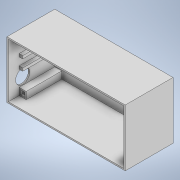
# Autodesk Inventor part: TimBoden
Saved by Autodesk Inventor 2022 (Build 260153000, 153)
## iProperties
Created: 2023-01-01
Part Number: TimBoden
Material: Generisch
Document SubType Name: Modeling
Designer: Joshua
Density: 1 g/cm^3
Appearance: Vorgabe
Author: Joshua
Autodesk Inventor part; units mm, degrees
ref_plane "YZ Plane" through (0, 0, 0) normal (1, 0, 0) x (0, 1, 0)
ref_plane "XZ Plane" through (0, 0, 0) normal (0, 1, 0) x (-1, 0, 0)
ref_plane "XY Plane" through (0, 0, 0) normal (0, 0, 1) x (1, 0, 0)
sketch "Skizze1" plane through (0, 0, 0) normal (0, 0, 1) x (1, 0, 0)
  line L0 (0, 0) -> (166, 0)
  line L1 (166, 0) -> (166, 80)
  line L2 (166, 80) -> (0, 80)
  line L3 (0, 80) -> (0, 0)
  dimension "d0" = 80
  dimension "d1" = 166
  constraints: 8 end point, 2 parallel, 1 horizontal, 1 perpendicular
  measures "d0" distance of L2.end L0.start
  measures "d1" distance of L1.end L2.end
extrude "Extrusion1" add sketch "Skizze1" along normal blind 2
sketch "Skizze2" plane through (0, 0, 2) normal (0, 0, 1) x (1, 0, 0)
  line L0 (0, 80) -> (0, 0) projected
  line L1 (166, 0) -> (166, 80) projected
  line L2 (0, 0) -> (166, 0)
  line L3 (166, 0) -> (166, 80)
  line L4 (166, 80) -> (0, 80)
  line L5 (0, 80) -> (0, 0)
  line L6 (2, 78) -> (164, 78)
  line L7 (164, 78) -> (164, 2)
  line L8 (164, 2) -> (2, 2)
  line L9 (2, 2) -> (2, 78)
  dimension "d4" = 2
  dimension "d6" = 2
  dimension "d7" = 2
  dimension "d8" = 2
  constraints: 16 end point, 4 parallel, 2 horizontal, 2 perpendicular
  measures "d4" distance between parallel lines of L0 L9
  measures "d6" distance between parallel lines of L4 L6
  measures "d7" distance between parallel lines of L1 L7
  measures "d8" distance between parallel lines of L2 L8
extrude "Extrusion2" add sketch "Skizze2" along normal blind 65
sketch "Skizze4" plane through (0, 0, 2) normal (0, 0, 1) x (1, 0, 0)
  line L0 (2, 2) -> (2, 78) projected
  line L1 (164, 2) -> (2, 2) projected
  line L2 (2, 78) -> (164, 78)
  line L3 (164, 78) -> (164, 2)
  line L4 (164, 2) -> (2, 2)
  line L5 (2, 2) -> (2, 78)
  line L6 (2, 68) -> (12, 68)
  line L7 (12, 68) -> (12, 78)
  line L8 (12, 78) -> (2, 78)
  line L9 (2, 78) -> (2, 68)
  line L10 (2, 2) -> (12, 2)
  line L11 (12, 2) -> (12, 12)
  line L12 (12, 12) -> (2, 12)
  line L13 (2, 12) -> (2, 2)
  line L14 (164, 78) -> (164, 2) projected
  line L15 (2, 78) -> (164, 78) projected
  line L16 (164, 68) -> (154, 68)
  line L17 (154, 68) -> (154, 78)
  line L18 (154, 78) -> (164, 78)
  line L19 (164, 78) -> (164, 68)
  line L20 (164, 2) -> (154, 2)
  line L21 (154, 2) -> (154, 12)
  line L22 (154, 12) -> (164, 12)
  line L23 (164, 12) -> (164, 2)
  point P0 (0, 0)
  point P1 (164, 12)
  point P2 (12, 2)
  point P3 (2, 68)
  dimension "d20" = 10
  dimension "d21" = 10
  dimension "d22" = 10
  dimension "d23" = 10
  dimension "d41" = 10
  dimension "d55" = 10
  constraints: 40 end point, 10 parallel, 5 horizontal, 5 perpendicular, 4 point on line
  measures "d20" distance of L6.end L7.end
  measures "d21" distance of L6.start L6.end
  measures "d22" distance of L10.end L11.end
  measures "d23" distance of L16.start L16.end
  measures "d41" distance of L11.end L12.end
  measures "d55" distance of L16.end L17.end
extrude "Extrusion3" add sketch "Skizze4" along normal blind 50 contours L0 L12 L11 L1 | L0 L2 L7 L6 | L21 L22 L3 L1 | L2 L3 L16 L17
sketch "Skizze5" plane through (0, 0, 2) normal (0, 0, 1) x (1, 0, 0)
  line L0 (2, 78) -> (164, 78) projected
  line L1 (2, 2) -> (2, 78) projected
  line L2 (2, 53) -> (7, 53)
  line L3 (7, 53) -> (7, 49)
  line L4 (7, 49) -> (2, 49)
  line L5 (2, 49) -> (2, 53)
  line L6 (2, 38) -> (7, 38)
  line L7 (7, 38) -> (7, 34)
  line L8 (7, 34) -> (2, 34)
  line L9 (2, 34) -> (2, 38)
  line L10 (164, 49) -> (159, 49)
  line L11 (159, 49) -> (159, 53)
  line L12 (159, 53) -> (164, 53)
  line L13 (164, 53) -> (164, 49)
  line L14 (164, 78) -> (164, 2) projected
  line L15 (164, 34) -> (159, 34)
  line L16 (159, 34) -> (159, 38)
  line L17 (159, 38) -> (164, 38)
  line L18 (164, 38) -> (164, 34)
  point P0 (0, 0)
  point P1 (2, 34)
  point P2 (2, 49)
  dimension "d30" = 11
  dimension "d31" = 4
  dimension "d32" = 4
  dimension "d33" = 5
  dimension "d34" = 25
  dimension "d37" = 5
  dimension "d38" = 0
  dimension "d58" = 25
  dimension "d59" = 4
  dimension "d60" = 11
  constraints: 32 end point, 8 parallel, 4 horizontal, 4 perpendicular, 4 point on line
  measures "d30" distance between parallel lines of L6 L4
  measures "d31" distance of L2.end L3.end
  measures "d32" distance of L6.end L7.end
  measures "d33" distance of L2.start L2.end
  measures "d34" distance between parallel lines of L0 L2
  measures "d37" distance of L11.end L12.end
  measures "d38" distance between parallel lines of L14 L13
  measures "d58" distance between parallel lines of L0 L12
  measures "d59" distance of L10.end L11.end
  measures "d60" distance between parallel lines of L10 L17
extrude "Extrusion4" add sketch "Skizze5" along normal blind 50
sketch "Skizze3" plane through (0, 0, 0) normal (-1, 0, 0) x (0, 0, 1)
  line L0 (0, 80) -> (67, 80) projected
  line L1 (52, 12) -> (2, 12) projected
  line L2 (2, 34) -> (52, 34) projected
  line L3 (2, 34) -> (2, 12) projected
  point P0 (0, 0)
  point P1 (47, 23)
  point P2 (67, 12)
  point P3 (67, 34)
  dimension "d52" = 11
  dimension "d53" = 11
  dimension "d54" = 45
  measures "d52" distance from line of L1 point (47, 23)
  measures "d53" distance from line of L2 point (47, 23)
  measures "d54" distance from line of L3 point (47, 23)
hole "Bohrung1" at (0, 23, 47) direction (1, 0, 0) diameter 20 depth 8 tip angle 118
sketch "Skizze6" plane through (0, 0, 52) normal (0, 0, 1) x (1, 0, 0)
  line L0 (4.15, 76.15) -> (9.85, 76.15)
  line L1 (9.85, 76.15) -> (9.85, 69.85)
  line L2 (9.85, 69.85) -> (4.15, 69.85)
  line L3 (4.15, 69.85) -> (4.15, 76.15)
  line L4 (2, 2) -> (2, 78) projected
  line L5 (2, 68) -> (12, 68) projected
  line L6 (4.15, 10.15) -> (9.85, 10.15)
  line L7 (9.85, 10.15) -> (9.85, 3.85)
  line L8 (9.85, 3.85) -> (4.15, 3.85)
  line L9 (4.15, 3.85) -> (4.15, 10.15)
  line L10 (12, 12) -> (2, 12) projected
  line L11 (156.15, 76.15) -> (161.85, 76.15)
  line L12 (161.85, 76.15) -> (161.85, 69.85)
  line L13 (161.85, 69.85) -> (156.15, 69.85)
  line L14 (156.15, 69.85) -> (156.15, 76.15)
  line L15 (154, 78) -> (154, 68) projected
  line L16 (156.15, 10.15) -> (161.85, 10.15)
  line L17 (161.85, 10.15) -> (161.85, 3.85)
  line L18 (161.85, 3.85) -> (156.15, 3.85)
  line L19 (156.15, 3.85) -> (156.15, 10.15)
  line L20 (2, 78) -> (164, 78) projected
  point P0 (0, 0)
  dimension "d42" = 5.7
  dimension "d43" = 6.3
  dimension "d44" = 2.15
  dimension "d45" = 1.85
  dimension "d46" = 6.3
  dimension "d47" = 1.85
  dimension "d48" = 5.7
  dimension "d49" = 2.15
  dimension "d56" = 1.85
  dimension "d57" = 6.3
  constraints: 32 end point, 8 parallel, 4 horizontal, 4 perpendicular
  measures "d42" distance of L0.start L0.end
  measures "d43" distance of L2.end L0.start
  measures "d44" distance between parallel lines of L4 L3
  measures "d45" distance between parallel lines of L5 L2
  measures "d46" distance of L8.end L6.start
  measures "d47" distance between parallel lines of L10 L6
  measures "d48" distance of L11.start L11.end
  measures "d49" distance between parallel lines of L15 L14
  measures "d56" distance between parallel lines of L20 L11
  measures "d57" distance of L13.end L11.start
extrude "Extrusion5" cut sketch "Skizze6" against normal blind 3
